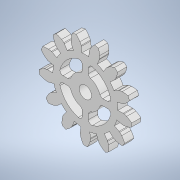
# Autodesk Inventor part: ｍ2歯数13ギアd3.99
Saved by Autodesk Inventor 2020.2 (Build 242310000, 310)
## iProperties
Created: 2020-02-11
Part Number: ｍ2歯数13ギアd3.99
Material: アルミニウム 2014-T4
Document SubType Name: Modeling
Designer: aoyam
Density: 2.8 g/cm^3
Appearance: サテン
Author: aoyam
Autodesk Inventor part; units mm, degrees
ref_plane "YZ Plane" through (0, 0, 0) normal (1, 0, 0) x (0, 1, 0)
ref_plane "XZ Plane" through (0, 0, 0) normal (0, 1, 0) x (-1, 0, 0)
ref_plane "XY Plane" through (0, 0, 0) normal (0, 0, 1) x (1, 0, 0)
sketch "スケッチ1" plane through (0, 0, 0) normal (0, 0, 1) x (1, 0, 0)
  arc A0 (149.8566, 117.4069) -> (149.7916, 117.1475) centre (151.2088, 116.9303) ccw
  arc A1 (150.243, 118.2214) -> (149.8566, 117.4069) centre (153.6231, 116.1188) ccw
  arc A2 (151.4709, 119.7028) -> (150.243, 118.2214) centre (156.2171, 114.5193) ccw
  arc A3 (147.2084, 117.1475) -> (147.1434, 117.4069) centre (145.7912, 116.9303) ccw
  arc A4 (147.1434, 117.4069) -> (146.757, 118.2214) centre (143.3769, 116.1188) ccw
  arc A5 (146.757, 118.2214) -> (145.5291, 119.7028) centre (140.7829, 114.5193) ccw
  arc A6 (149.6101, 115.4411) -> (147.3899, 115.4411) centre (148.5, 105) ccw
  arc A7 (145.5291, 119.7028) -> (144.2978, 119.3994) centre (148.5, 105) ccw
  line L0 (149.6101, 115.4411) -> (149.7916, 117.1475)
  line L1 (147.3899, 115.4411) -> (147.2084, 117.1475)
  line L2 (131.5, 105) -> (165.5, 105)
  line L3 (148.5, 88) -> (148.5, 122)
  line L4 (183.5, 120) -> (253.5, 120)
  line L5 (183.5, 112) -> (253.5, 112)
  line L6 (183.5, 104) -> (253.5, 104)
  line L7 (183.5, 96) -> (253.5, 96)
  line L8 (183.5, 88) -> (253.5, 88)
  line L9 (183.5, 80) -> (253.5, 80)
  line L10 (183.5, 72) -> (253.5, 72)
  line L11 (183.5, 64) -> (253.5, 64)
  line L12 (183.5, 56) -> (253.5, 56)
  line L13 (183.5, 48) -> (253.5, 48)
  line L14 (183.5, 40) -> (253.5, 40)
  line L15 (183.5, 32) -> (253.5, 32)
  line L16 (183.5, 24) -> (253.5, 24)
  line L17 (183.5, 120) -> (183.5, 24)
  line L18 (253.5, 120) -> (253.5, 24)
  line L19 (218.5, 112) -> (218.5, 24)
  arc A8 (143.9354, 116.6162) -> (143.9984, 116.3563) centre (145.3542, 116.8225) ccw
  line L20 (144.6307, 114.7611) -> (143.9984, 116.3563)
  arc A9 (143.8991, 117.517) -> (143.9354, 116.6162) centre (147.8691, 117.226) ccw
  arc A10 (144.2978, 119.3994) -> (143.8991, 117.517) centre (150.9093, 117.0153) ccw
  arc A11 (144.6307, 114.7611) -> (142.6648, 113.7293) centre (148.5, 105) ccw
  line L21 (142.6648, 113.7293) -> (141.7111, 115.1559)
  arc A12 (141.7111, 115.1559) -> (141.5331, 115.3553) centre (140.5572, 114.3049) ccw
  arc A13 (141.5331, 115.3553) -> (140.8123, 115.897) centre (138.7966, 112.4644) ccw
  arc A14 (140.8123, 115.897) -> (139.0366, 116.6381) centre (137.2429, 109.8426) ccw
  arc A15 (139.0366, 116.6381) -> (138.0875, 115.7972) centre (148.5, 105) ccw
  arc A16 (139.0599, 113.1643) -> (139.2365, 112.9635) centre (140.2203, 114.0064) ccw
  line L22 (140.5377, 111.8449) -> (139.2365, 112.9635)
  arc A17 (138.6091, 113.9451) -> (139.0599, 113.1643) centre (142.2596, 115.5324) ccw
  arc A18 (138.0875, 115.7972) -> (138.6091, 113.9451) centre (145.0496, 116.7587) ccw
  arc A19 (140.5377, 111.8449) -> (139.2765, 110.0176) centre (148.5, 105) ccw
  line L23 (139.2765, 110.0176) -> (137.7691, 110.8376)
  arc A20 (137.7691, 110.8376) -> (137.5187, 110.9315) centre (137.1428, 109.5479) ccw
  arc A21 (137.5187, 110.9315) -> (136.6288, 111.0762) centre (136.4392, 107.1) ccw
  arc A22 (136.6288, 111.0762) -> (134.7121, 110.9072) centre (136.2819, 104.0565) ccw
  arc A23 (134.7121, 110.9072) -> (134.2625, 109.7215) centre (148.5, 105) ccw
  arc A24 (136.3471, 107.8422) -> (136.5967, 107.7464) centre (136.9832, 109.127) ccw
  line L24 (138.2688, 107.3606) -> (136.5967, 107.7464)
  arc A25 (135.585, 108.324) -> (136.3471, 107.8422) centre (138.0798, 111.426) ccw
  arc A26 (134.2625, 109.7215) -> (135.585, 108.324) centre (139.9803, 113.8083) ccw
  arc A27 (138.2688, 107.3606) -> (138.0012, 105.1565) centre (148.5, 105) ccw
  line L25 (138.0012, 105.1565) -> (136.2854, 105.1821)
  arc A28 (136.2854, 105.1821) -> (136.0201, 105.1488) centre (136.3302, 103.749) ccw
  arc A29 (136.0201, 105.1488) -> (135.1649, 104.8633) centre (136.8447, 101.2545) ccw
  arc A30 (135.1649, 104.8633) -> (133.5462, 103.823) centre (138.1199, 98.4866) ccw
  arc A31 (133.5462, 103.823) -> (133.6991, 102.5641) centre (148.5, 105) ccw
  arc A32 (136.4183, 101.8689) -> (136.6839, 101.9001) centre (136.3845, 103.3022) ccw
  line L26 (138.3437, 102.3355) -> (136.6839, 101.9001)
  arc A33 (135.5196, 101.9414) -> (136.4183, 101.8689) centre (136.2871, 105.8474) ccw
  arc A34 (133.6991, 102.5641) -> (135.5196, 101.9414) centre (136.8627, 108.84) ccw
  arc A35 (138.3437, 102.3355) -> (139.131, 100.2595) centre (148.5, 105) ccw
  line L27 (139.131, 100.2595) -> (137.5999, 99.4848)
  arc A36 (137.5999, 99.4848) -> (137.3804, 99.3321) centre (138.3055, 98.2367) ccw
  arc A37 (137.3804, 99.3321) -> (136.7558, 98.6818) centre (139.9204, 96.2671) ccw
  arc A38 (136.7558, 98.6818) -> (135.8061, 97.0085) centre (142.3358, 94.4087) ccw
  arc A39 (135.8061, 97.0085) -> (136.5265, 95.9648) centre (148.5, 105) ccw
  arc A40 (139.2573, 96.6129) -> (139.4779, 96.7639) centre (138.5612, 97.8663) ccw
  line L28 (140.7453, 97.9209) -> (139.4779, 96.7639)
  arc A41 (138.4279, 96.2594) -> (139.2573, 96.6129) centre (137.2922, 100.0747) ccw
  arc A42 (136.5265, 95.9648) -> (138.4279, 96.2594) centre (136.4111, 102.9921) ccw
  arc A43 (140.7453, 97.9209) -> (142.4072, 96.4485) centre (148.5, 105) ccw
  line L29 (142.4072, 96.4485) -> (141.4115, 95.051)
  arc A44 (141.4115, 95.051) -> (141.2881, 94.8138) centre (142.6163, 94.2738) ccw
  arc A45 (141.2881, 94.8138) -> (141.0372, 93.9478) centre (144.9616, 93.2802) ccw
  arc A46 (141.0372, 93.9478) -> (140.974, 92.0247) centre (147.9639, 92.7573) ccw
  arc A47 (140.974, 92.0247) -> (142.0968, 91.4354) centre (148.5, 105) ccw
  arc A48 (144.2137, 93.2783) -> (144.3389, 93.5145) centre (143.0149, 94.0647) ccw
  line L30 (144.9234, 95.1279) -> (144.3389, 93.5145)
  arc A49 (143.6435, 92.5799) -> (144.2137, 93.2783) centre (140.8649, 95.4303) ccw
  arc A50 (142.0968, 91.4354) -> (143.6435, 92.5799) centre (138.729, 97.6041) ccw
  arc A51 (144.9234, 95.1279) -> (147.0792, 94.5966) centre (148.5, 105) ccw
  line L31 (147.0792, 94.5966) -> (146.8469, 92.8964)
  arc A52 (146.8469, 92.8964) -> (146.848, 92.629) centre (148.2749, 92.7682) ccw
  arc A53 (146.848, 92.629) -> (147.0283, 91.7456) centre (150.8133, 92.9783) ccw
  arc A54 (147.0283, 91.7456) -> (147.8659, 90.0134) centre (153.7148, 93.9104) ccw
  arc A55 (147.8659, 90.0134) -> (149.1341, 90.0134) centre (148.5, 105) ccw
  arc A56 (150.152, 92.629) -> (150.1531, 92.8964) centre (148.7251, 92.7682) ccw
  line L32 (149.9208, 94.5966) -> (150.1531, 92.8964)
  arc A57 (149.9717, 91.7456) -> (150.152, 92.629) centre (146.1867, 92.9783) ccw
  arc A58 (149.1341, 90.0134) -> (149.9717, 91.7456) centre (143.2852, 93.9104) ccw
  arc A59 (149.9208, 94.5966) -> (152.0766, 95.1279) centre (148.5, 105) ccw
  line L33 (152.0766, 95.1279) -> (152.6611, 93.5145)
  arc A60 (152.6611, 93.5145) -> (152.7863, 93.2783) centre (153.9851, 94.0647) ccw
  arc A61 (152.7863, 93.2783) -> (153.3565, 92.5799) centre (156.1351, 95.4303) ccw
  arc A62 (153.3565, 92.5799) -> (154.9032, 91.4354) centre (158.271, 97.6041) ccw
  arc A63 (154.9032, 91.4354) -> (156.026, 92.0247) centre (148.5, 105) ccw
  arc A64 (155.7119, 94.8138) -> (155.5885, 95.051) centre (154.3837, 94.2738) ccw
  line L34 (154.5928, 96.4485) -> (155.5885, 95.051)
  arc A65 (155.9628, 93.9478) -> (155.7119, 94.8138) centre (152.0384, 93.2802) ccw
  arc A66 (156.026, 92.0247) -> (155.9628, 93.9478) centre (149.0361, 92.7573) ccw
  arc A67 (154.5928, 96.4485) -> (156.2547, 97.9209) centre (148.5, 105) ccw
  line L35 (156.2547, 97.9209) -> (157.5221, 96.7639)
  arc A68 (157.5221, 96.7639) -> (157.7427, 96.6129) centre (158.4388, 97.8663) ccw
  arc A69 (157.7427, 96.6129) -> (158.5721, 96.2594) centre (159.7078, 100.0747) ccw
  arc A70 (158.5721, 96.2594) -> (160.4735, 95.9648) centre (160.5889, 102.9921) ccw
  arc A71 (160.4735, 95.9648) -> (161.1939, 97.0085) centre (148.5, 105) ccw
  arc A72 (159.6196, 99.3321) -> (159.4001, 99.4848) centre (158.6945, 98.2367) ccw
  line L36 (157.869, 100.2595) -> (159.4001, 99.4848)
  arc A73 (160.2442, 98.6818) -> (159.6196, 99.3321) centre (157.0796, 96.2671) ccw
  arc A74 (161.1939, 97.0085) -> (160.2442, 98.6818) centre (154.6642, 94.4087) ccw
  arc A75 (157.869, 100.2595) -> (158.6563, 102.3355) centre (148.5, 105) ccw
  line L37 (158.6563, 102.3355) -> (160.3161, 101.9001)
  arc A76 (160.3161, 101.9001) -> (160.5817, 101.8689) centre (160.6155, 103.3022) ccw
  arc A77 (160.5817, 101.8689) -> (161.4804, 101.9414) centre (160.7129, 105.8474) ccw
  arc A78 (161.4804, 101.9414) -> (163.3009, 102.5641) centre (160.1373, 108.84) ccw
  arc A79 (163.3009, 102.5641) -> (163.4538, 103.823) centre (148.5, 105) ccw
  arc A80 (160.9799, 105.1488) -> (160.7146, 105.1821) centre (160.6698, 103.749) ccw
  line L38 (158.9988, 105.1565) -> (160.7146, 105.1821)
  arc A81 (161.8351, 104.8633) -> (160.9799, 105.1488) centre (160.1553, 101.2545) ccw
  arc A82 (163.4538, 103.823) -> (161.8351, 104.8633) centre (158.8801, 98.4866) ccw
  arc A83 (158.9988, 105.1565) -> (158.7312, 107.3606) centre (148.5, 105) ccw
  line L39 (158.7312, 107.3606) -> (160.4033, 107.7464)
  arc A84 (160.4033, 107.7464) -> (160.6529, 107.8422) centre (160.0168, 109.127) ccw
  arc A85 (160.6529, 107.8422) -> (161.415, 108.324) centre (158.9202, 111.426) ccw
  arc A86 (161.415, 108.324) -> (162.7375, 109.7215) centre (157.0197, 113.8083) ccw
  arc A87 (162.7375, 109.7215) -> (162.2879, 110.9072) centre (148.5, 105) ccw
  arc A88 (159.4813, 110.9315) -> (159.2309, 110.8376) centre (159.8572, 109.5479) ccw
  line L40 (157.7235, 110.0176) -> (159.2309, 110.8376)
  arc A89 (160.3712, 111.0762) -> (159.4813, 110.9315) centre (160.5608, 107.1) ccw
  arc A90 (162.2879, 110.9072) -> (160.3712, 111.0762) centre (160.7181, 104.0565) ccw
  arc A91 (157.7235, 110.0176) -> (156.4623, 111.8449) centre (148.5, 105) ccw
  line L41 (156.4623, 111.8449) -> (157.7635, 112.9635)
  arc A92 (157.7635, 112.9635) -> (157.9401, 113.1643) centre (156.7797, 114.0064) ccw
  arc A93 (157.9401, 113.1643) -> (158.3909, 113.9451) centre (154.7404, 115.5324) ccw
  arc A94 (158.3909, 113.9451) -> (158.9125, 115.7972) centre (151.9504, 116.7587) ccw
  arc A95 (158.9125, 115.7972) -> (157.9634, 116.6381) centre (148.5, 105) ccw
  arc A96 (155.4669, 115.3553) -> (155.2889, 115.1559) centre (156.4428, 114.3049) ccw
  line L42 (154.3352, 113.7293) -> (155.2889, 115.1559)
  arc A97 (156.1877, 115.897) -> (155.4669, 115.3553) centre (158.2034, 112.4644) ccw
  arc A98 (157.9634, 116.6381) -> (156.1877, 115.897) centre (159.7571, 109.8426) ccw
  arc A99 (154.3352, 113.7293) -> (152.3693, 114.7611) centre (148.5, 105) ccw
  line L43 (152.3693, 114.7611) -> (153.0016, 116.3563)
  arc A100 (153.0016, 116.3563) -> (153.0646, 116.6162) centre (151.6458, 116.8225) ccw
  arc A101 (153.0646, 116.6162) -> (153.1009, 117.517) centre (149.1309, 117.226) ccw
  arc A102 (153.1009, 117.517) -> (152.7022, 119.3994) centre (146.0907, 117.0153) ccw
  arc A103 (152.7022, 119.3994) -> (151.4709, 119.7028) centre (148.5, 105) ccw
  circle A104 centre (148.5, 105) radius 5
  circle A105 centre (148.5, 105) radius 5.6
  circle A106 centre (146.3889, 112.4569) radius 1.5
  circle A107 centre (148.5, 105) radius 10.5
  circle A108 centre (148.5, 105) radius 7.75 construction
  circle A109 centre (141.0431, 102.8889) radius 1.5
  circle A110 centre (150.6111, 97.5431) radius 1.5
  circle A111 centre (155.9569, 107.1111) radius 1.5
  circle A112 centre (148.5, 105) radius 1.99
  point P0 (0, 0)
  point P1 (189.5, 114)
  point P2 (192, 106)
  point P3 (192, 98)
  point P4 (189.5, 90)
  point P5 (192, 82)
  point P6 (187, 74)
  point P7 (189.5, 66)
  point P8 (189.5, 58)
  point P9 (189.5, 50)
  point P10 (192, 42)
  point P11 (192, 34)
  point P12 (189.5, 26)
  point P13 (219.5, 106)
  point P14 (234.5, 98)
  point P15 (235.75, 90)
  point P16 (232, 82)
  point P17 (234.5, 74)
  point P18 (229.5, 66)
  point P19 (234.5, 58)
  point P20 (234.5, 50)
  point P21 (229.5, 42)
  point P22 (237, 34)
  point P23 (237, 26)
  point P24 (149.5, 135.5)
  point P25 (149.5, 129.5)
  point P26 (166.75, 135.5)
  point P27 (167.8125, 129.5)
  point P28 (140.5997, 120.0528)
  point P29 (134.5093, 114.6571)
  point P30 (131.6239, 107.0491)
  point P31 (132.6047, 98.9717)
  point P32 (137.2269, 92.2753)
  point P33 (144.4316, 88.494)
  point P34 (152.5684, 88.494)
  point P35 (159.7731, 92.2753)
  point P36 (164.3953, 98.9717)
  point P37 (165.3761, 107.0491)
  point P38 (162.4907, 114.6571)
  point P39 (156.4003, 120.0528)
  point P40 (149.1341, 90.0134)
  point P41 (149.9717, 91.7456)
  point P42 (150.152, 92.629)
  point P43 (149.9208, 94.5966)
  point P44 (152.7863, 93.2783)
  point P45 (153.3565, 92.5799)
  point P46 (154.9032, 91.4354)
  point P47 (156.026, 92.0247)
  point P48 (155.9628, 93.9478)
  point P49 (154.5928, 96.4485)
  point P50 (157.5221, 96.7639)
  point P51 (157.7427, 96.6129)
  point P52 (158.5721, 96.2594)
  point P53 (160.4735, 95.9648)
  point P54 (161.1939, 97.0085)
  point P55 (160.2442, 98.6818)
  point P56 (160.3161, 101.9001)
  point P57 (160.5817, 101.8689)
  point P58 (161.4804, 101.9414)
  point P59 (161.8351, 104.8633)
  point P60 (160.6529, 107.8422)
  point P61 (162.7375, 109.7215)
  point P62 (162.2879, 110.9072)
  point P63 (160.3712, 111.0762)
  point P64 (159.4813, 110.9315)
  point P65 (157.7235, 110.0176)
  point P66 (157.7635, 112.9635)
  point P67 (157.9401, 113.1643)
  point P68 (158.3909, 113.9451)
  point P69 (158.9125, 115.7972)
  point P70 (154.3352, 113.7293)
  point P71 (153.0016, 116.3563)
  point P72 (152.7022, 119.3994)
  point P73 (151.4709, 119.7028)
  point P74 (150.243, 118.2214)
  point P75 (149.8566, 117.4069)
  point P76 (147.3899, 115.4411)
  point P77 (146.757, 118.2214)
  point P78 (144.2978, 119.3994)
  point P79 (143.8991, 117.517)
  point P80 (144.6307, 114.7611)
  point P81 (140.8123, 115.897)
  point P82 (139.0366, 116.6381)
  point P83 (138.0875, 115.7972)
  point P84 (138.6091, 113.9451)
  point P85 (139.0599, 113.1643)
  point P86 (140.5377, 111.8449)
  point P87 (137.7691, 110.8376)
  point P88 (137.5187, 110.9315)
  point P89 (136.6288, 111.0762)
  point P90 (134.7121, 110.9072)
  point P91 (134.2625, 109.7215)
  point P92 (135.585, 108.324)
  point P93 (138.2688, 107.3606)
  point P94 (133.5462, 103.823)
  point P95 (133.6991, 102.5641)
  point P96 (135.5196, 101.9414)
  point P97 (136.4183, 101.8689)
  point P98 (138.3437, 102.3355)
  point P99 (137.5999, 99.4848)
  point P100 (137.3804, 99.3321)
  point P101 (142.0968, 91.4354)
  point P102 (144.2137, 93.2783)
  point P103 (147.8659, 90.0134)
  dimension "d11" = 15.5
  dimension "d2" = 360
  dimension "d4" = 10
  dimension "d7" = 0.6
  dimension "d10" = 3
  dimension "d14" = 360
  dimension "d16" = 3.98
  constraints: 208 point on circle, 112 centre point, 88 end point, 5 coincident, 1 concentric, 1 midpoint, 545 other
  measures "d4" diameter of A104
  measures "d7" radial gap between concentric circles of A104 A105
  measures "d10" diameter of A106
  measures "d16" diameter of A112
extrude "押し出し1" add sketch "スケッチ1" along normal blind 3 contours A1 A2 A103 A102 A101 A100 L43 A107 L0 A0 | A107 A99 A91 A83 L2 A105 L3 A6 | L3 A105 L2 A107 A27 A19 A11 A6 | A107 L20 A8 A9 A10 A7 A5 A4 A3 L1 | A105 L2 A104 L3 | L3 A104 L2 A105 | L42 A96 A97 A98 A95 A94 A93 A92 L41 A107 | A104 L2 A112 L3 | L3 A112 L2 A104 | A105 L3 A104 L2 | L2 A107 A75 A67 A59 L3 A105 | A105 L3 A107 A51 A43 A35 L2 | L2 A104 L3 A105 | A107 L22 A16 A17 A18 A15 A14 A13 A12 L21 | A104 L3 A112 L2 | L2 A112 L3 A104 | A107 L38 A80 A81 L2 | L2 A81 A82 A79 A78 A77 A76 L37 A107 | A107 L26 A32 A33 A34 A31 A30 A29 L2 | L2 A29 A28 L25 A107 | L40 A88 A89 A90 A87 A86 A85 A84 L39 A107 | A107 L32 A56 A57 A58 A55 L3 | L3 A55 A54 A53 A52 L31 A107 | A107 L24 A24 A25 A26 A23 A22 A21 A20 L23 | L36 A72 A73 A74 A71 A70 A69 A68 L35 A107 | A107 L28 A40 A41 A42 A39 A38 A37 A36 L27 | L30 A48 A49 A50 A47 A46 A45 A44 L29 A107 | A107 L34 A64 A65 A66 A63 A62 A61 A60 L33 | A106 | A109 | A110 | A111
sketch "スケッチ2" plane through (0, 0, 3) normal (0, 0, 1) x (1, 0, 0)
  circle A0 centre (148.5, 105) radius 1.99 projected
  circle A1 centre (148.5, 105) radius 10.5
  circle A2 centre (148.5, 105) radius 8.5
  circle A3 centre (148.5, 105) radius 4.99
  line L0 (148.5, 105) -> (153.49, 105) construction
  line L1 (153.49, 105) -> (157, 105) construction
  line L2 (153.49, 105) -> (157, 105) construction
  line L3 (153.49, 104) -> (154.1498, 104)
  line L4 (156.941, 106) -> (155.7218, 106)
  arc A4 (153.49, 106) -> (153.3898, 105.995) centre (153.49, 105) ccw
  arc A5 (153.3898, 104.005) -> (153.49, 104) centre (153.49, 105) ccw
  arc A6 (153.2027, 106.6689) -> (154.1498, 106) centre (154.1498, 107.005) ccw
  arc A7 (154.1498, 104) -> (153.2027, 103.3311) centre (154.1498, 102.995) ccw
  arc A8 (155.7218, 106) -> (156.6902, 107.2738) centre (155.7218, 107.005) ccw
  arc A9 (156.6902, 102.7262) -> (155.7218, 104) centre (155.7218, 102.995) ccw
  line L5 (155.7218, 106) -> (154.1498, 106)
  line L6 (154.1498, 106) -> (153.49, 106)
  line L7 (154.1498, 104) -> (156.941, 104)
  arc A10 (146.8311, 109.7027) -> (147.5, 110.6498) centre (146.495, 110.6498) ccw
  arc A11 (149.5, 110.6498) -> (150.1689, 109.7027) centre (150.505, 110.6498) ccw
  line L8 (149.5, 110.6498) -> (149.5, 113.441)
  line L9 (147.5, 112.2218) -> (147.5, 110.6498)
  arc A12 (147.5, 112.2218) -> (146.2262, 113.1902) centre (146.495, 112.2218) ccw
  arc A13 (150.7738, 113.1902) -> (149.5, 112.2218) centre (150.505, 112.2218) ccw
  arc A14 (143.7973, 103.3311) -> (142.8502, 104) centre (142.8502, 102.995) ccw
  arc A15 (142.8502, 106) -> (143.7973, 106.6689) centre (142.8502, 107.005) ccw
  line L10 (142.8502, 106) -> (140.059, 106)
  line L11 (141.2782, 104) -> (142.8502, 104)
  arc A16 (141.2782, 104) -> (140.3098, 102.7262) centre (141.2782, 102.995) ccw
  arc A17 (140.3098, 107.2738) -> (141.2782, 106) centre (141.2782, 107.005) ccw
  arc A18 (150.1689, 100.2973) -> (149.5, 99.3502) centre (150.505, 99.3502) ccw
  arc A19 (147.5, 99.3502) -> (146.8311, 100.2973) centre (146.495, 99.3502) ccw
  line L12 (147.5, 99.3502) -> (147.5, 96.559)
  line L13 (149.5, 97.7782) -> (149.5, 99.3502)
  arc A20 (149.5, 97.7782) -> (150.7738, 96.8098) centre (150.505, 97.7782) ccw
  arc A21 (146.2262, 96.8098) -> (147.5, 97.7782) centre (146.495, 97.7782) ccw
  point P0 (0, 0)
  point P1 (155.245, 105)
  dimension "d17" = 21
  dimension "d18" = 2
  dimension "d19" = 3
  dimension "d21" = 2
  dimension "d22" = 2.01
  dimension "d23" = 2.01
  dimension "d24" = 2.01
  dimension "d27" = 360
  constraints: 45 point on circle, 30 end point, 21 centre point, 16 tangent, 6 parallel, 5 horizontal, 3 symmetric about line, 1 coincident, 1 collinear, 1 midpoint, 1 point on line, 78 other
  measures "d17" diameter of A1
  measures "d18" radial gap between concentric circles of A1 A2
  measures "d19" radial gap between concentric circles of A0 A3
  measures "d21" distance between parallel lines of L3 L4
  measures "d22" diameter of A6
  measures "d23" diameter of A7
  measures "d24" diameter of A8
extrude "押し出し3" cut sketch "スケッチ2" against normal blind 3 contours A8 L5 A6 A3 A11 L8 A13 A2 | A2 A20 L13 A18 A3 A7 L7 A9 | A12 L9 A10 A3 A15 L10 A17 A2 | A2 A16 L11 A14 A3 A19 L12 A21
